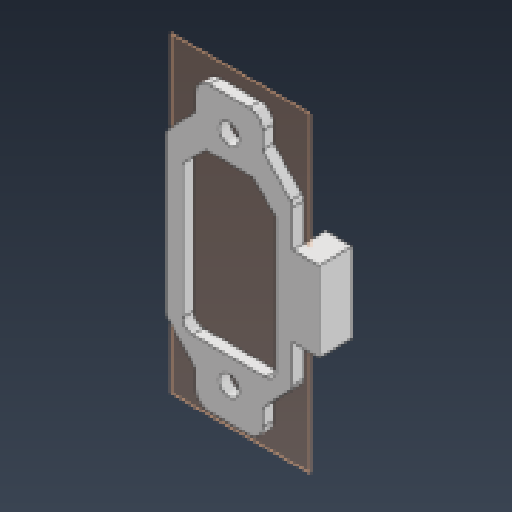
# Autodesk Inventor part: 4
Saved by Autodesk Inventor 2023 (Build 270158000, 158)
## iProperties
Created: 2026-01-23
Part Number: 4
Material: Generic
Document SubType Name: Modeling
Designer: szymo
Density: 1 g/cm^3
Appearance: Default
Author: szymo
Autodesk Inventor part; units mm, degrees
ref_plane "YZ Plane" through (0, 0, 0) normal (1, 0, 0) x (0, 1, 0)
ref_plane "XZ Plane" through (0, 0, 0) normal (0, 1, 0) x (-1, 0, 0)
ref_plane "XY Plane" through (0, 0, 0) normal (0, 0, 1) x (1, 0, 0)
ref_plane "Work Plane1" through (0, 0, 0) normal (0, 0, 1) x (1, 0, 0)
sketch "Sketch1" plane through (0, 0, 0) normal (0, 0, 1) x (1, 0, 0)
  line L0 (9.226, 12.2893) -> (5, 16.75) projected
  line L1 (5, 16.75) -> (5, 19.25) projected
  arc A0 (5, 19.25) -> (3, 21.25) centre (3, 19.25) ccw projected
  line L2 (3, 21.25) -> (-3, 21.25) projected
  arc A1 (-3, 21.25) -> (-5, 19.25) centre (-3, 19.25) ccw projected
  line L3 (-5, 19.25) -> (-5, 16.75) projected
  line L4 (-5, 16.75) -> (-9.226, 12.2893) projected
  arc A2 (-9.226, 12.2893) -> (-9.5, 11.6015) centre (-8.5, 11.6015) ccw projected
  line L5 (-9.5, 11.6015) -> (-9.5, -11.6015) projected
  arc A3 (-9.5, -11.6015) -> (-9.226, -12.2893) centre (-8.5, -11.6015) ccw projected
  line L6 (-5, -16.75) -> (-9.226, -12.2893) projected
  line L7 (-5, -19.25) -> (-5, -16.75) projected
  arc A4 (-5, -19.25) -> (-3, -21.25) centre (-3, -19.25) ccw projected
  line L8 (3, -21.25) -> (-3, -21.25) projected
  arc A5 (3, -21.25) -> (5, -19.25) centre (3, -19.25) ccw projected
  line L9 (5, -16.75) -> (5, -19.25) projected
  line L10 (9.226, -12.2893) -> (5, -16.75) projected
  arc A6 (9.226, -12.2893) -> (9.5, -11.6015) centre (8.5, -11.6015) ccw projected
  line L11 (9.5, -11.6015) -> (9.5, 11.6015) projected
  arc A7 (9.5, 11.6015) -> (9.226, 12.2893) centre (8.5, 11.6015) ccw projected
  circle A8 centre (0, -16.35) radius 1.5 projected
  circle A9 centre (0, 16.35) radius 1.5 projected
  line L12 (-7, 9) -> (-7, -11) projected
  line L13 (-7, 9) -> (-3.5, 12.5) projected
  line L14 (3.5, 12.5) -> (-3.5, 12.5) projected
  line L15 (3.5, 12.5) -> (7, 9) projected
  line L16 (7, -11) -> (7, 9) projected
  arc A10 (5.5, -12.5) -> (7, -11) centre (5.5, -11) ccw projected
  line L17 (-5.5, -12.5) -> (5.5, -12.5) projected
  arc A11 (-7, -11) -> (-5.5, -12.5) centre (-5.5, -11) ccw projected
  point P0 (0, 0)
extrude "Extrusion1" add sketch "Sketch1" along normal blind 1.7
sketch "Sketch2" plane through (0, 0, 1.7) normal (0, 0, 1) x (1, 0, 0)
  line L0 (9.5, -11.6015) -> (9.5, 11.6015) projected
  arc A0 (9.5, 11.6015) -> (9.226, 12.2893) centre (8.5, 11.6015) ccw projected
  line L1 (9.226, 12.2893) -> (5, 16.75) projected
  line L2 (5, 16.75) -> (5, 19.25) projected
  arc A1 (5, 19.25) -> (3, 21.25) centre (3, 19.25) ccw projected
  line L3 (3, 21.25) -> (-3, 21.25) projected
  arc A2 (-3, 21.25) -> (-5, 19.25) centre (-3, 19.25) ccw projected
  line L4 (-5, 19.25) -> (-5, 16.75) projected
  line L5 (-5, 16.75) -> (-9.226, 12.2893) projected
  arc A3 (-9.226, 12.2893) -> (-9.5, 11.6015) centre (-8.5, 11.6015) ccw projected
  line L6 (-9.5, 11.6015) -> (-9.5, -11.6015) projected
  arc A4 (-9.5, -11.6015) -> (-9.226, -12.2893) centre (-8.5, -11.6015) ccw projected
  line L7 (-9.226, -12.2893) -> (-5, -16.75) projected
  line L8 (-5, -16.75) -> (-5, -19.25) projected
  arc A5 (-5, -19.25) -> (-3, -21.25) centre (-3, -19.25) ccw projected
  line L9 (-3, -21.25) -> (3, -21.25) projected
  arc A6 (3, -21.25) -> (5, -19.25) centre (3, -19.25) ccw projected
  line L10 (5, -19.25) -> (5, -16.75) projected
  line L11 (5, -16.75) -> (9.226, -12.2893) projected
  arc A7 (9.226, -12.2893) -> (9.5, -11.6015) centre (8.5, -11.6015) ccw projected
  circle A8 centre (0, -16.35) radius 1.5 projected
  circle A9 centre (0, 16.35) radius 1.5 projected
  line L12 (3.5, 12.5) -> (7, 9) projected
  line L13 (7, 9) -> (7, -11) projected
  arc A10 (5.5, -12.5) -> (7, -11) centre (5.5, -11) ccw projected
  line L14 (5.5, -12.5) -> (-5.5, -12.5) projected
  arc A11 (-7, -11) -> (-5.5, -12.5) centre (-5.5, -11) ccw projected
  line L15 (-7, -11) -> (-7, 9) projected
  line L16 (-7, 9) -> (-3.5, 12.5) projected
  line L17 (-3.5, 12.5) -> (3.5, 12.5) projected
  line L18 (5.5, -6) -> (13.5, -6)
  line L19 (13.5, -6) -> (13.5, 6)
  line L20 (13.5, 6) -> (5.5, 6)
  line L21 (5.5, 6) -> (5.5, -6)
  line L22 (5.5, -6) -> (13.5, 6) construction
  line L23 (13.5, -6) -> (5.5, 6) construction
  point P0 (0, 0)
  point P1 (9.5, 0)
  point P2 (9.5, 6)
  point P3 (9.5, -6)
  dimension "d2" = 12
  dimension "d3" = 4
  constraints: 12 end point, 3 midpoint, 2 parallel, 1 horizontal, 1 perpendicular
  measures "d2" distance of L18.end L19.end
  measures "d3" distance between parallel lines of L19 L0
ref_plane "Work Plane2" through (-9.5, -21.25, -3.3) normal (0, 0, -1) x (0, 1, 0)
extrude "Extrusion2" add sketch "Sketch2" against normal up to surface (5 mm away) contours L0 L20 L19 L18
body "Solid1"
